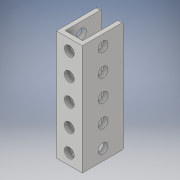
# Autodesk Inventor part: Mini Channel 5 Holes
Saved by Autodesk Inventor 2019 (Build 230136000, 136)
## iProperties
Created: 2016-08-22
Part Number: Mini Channel 5 Holes
Material: Generic
Description: STEP AP203
Document SubType Name: Modeling
Designer: mrhftc
Density: 1 g/cm^3
Appearance: Default
Sending System: SolidWorks 2014
Preprocessor: SwSTEP 2.0
Title: 585380.STEP
Revision Number: ANY
Autodesk Inventor part; units mm, degrees
ref_plane "YZ Plane" through (0, 0, 0) normal (1, 0, 0) x (0, 1, 0)
ref_plane "Work Plane1" through (4.699, 0, 1.524) normal (1, 0, 0) x (0, 0, -1)
sketch "Sketch1" plane through (4.699, 0, 1.524) normal (1, 0, 0) x (0, 0, -1)
  line L0 (-11.9322, 40.005) -> (-26.9436, 40.005)
  line L1 (-26.9436, 40.005) -> (-26.9436, 0)
  line L2 (-26.9436, 0) -> (-11.9322, 0)
  line L3 (-11.9322, 0) -> (-11.9322, 40.005)
  circle A0 centre (-19.4379, 20.0025) radius 1.778
  circle A1 centre (-19.4379, 28.0035) radius 1.778
  circle A2 centre (-19.4379, 36.0045) radius 1.778
  line L4 (-11.9322, 20.0025) -> (-25.268, 20.0025)
  circle A3 centre (-19.4379, 12.0015) radius 1.778
  circle A4 centre (-19.4379, 4.0005) radius 1.778
  point P0 (1.524, 0)
  dimension "d0" = 40.005
  dimension "d1" = 15.0114
  dimension "d2" = 3.556
  dimension "d3" = 3.556
  dimension "d4" = 3.556
  dimension "d6" = 8.001
  dimension "d7" = 8.001
  constraints: 10 end point, 5 centre point, 2 horizontal, 2 parallel, 2 symmetric about line, 1 midpoint, 1 perpendicular, 2 other
  measures "d0" distance between parallel lines of L2 L0
  measures "d1" distance between parallel lines of L1 L3
  measures "d2" diameter of A0
  measures "d3" diameter of A2
  measures "d4" diameter of A1
  measures "d6" distance of A0.centre A1.centre
  measures "d7" distance of A1.centre A2.centre
extrude "Extrusion1" add sketch "Sketch1" along normal blind 9.398
ref_plane "Work Plane2" through (4.699, 0, 13.4562) normal (0, -1, 0) x (1, 0, 0)
sketch "Sketch2" plane through (4.699, 0, 13.4562) normal (0, -1, 0) x (1, 0, 0)
  line L0 (0, 0) -> (9.398, 0) construction
  line L1 (9.398, 15.0114) -> (9.398, 0) construction
  line L2 (7.874, 13.335) -> (1.524, 13.335)
  line L3 (1.524, 13.335) -> (1.524, 0)
  line L4 (1.524, 0) -> (7.874, 0)
  line L5 (7.874, 0) -> (7.874, 13.335)
  line L6 (0, 0) -> (9.398, 0) construction
  point P0 (-4.699, -13.4562)
  dimension "d10" = 6.35
  dimension "d11" = 1.524
  dimension "d13" = 13.335
  constraints: 8 end point, 2 parallel, 1 horizontal, 1 perpendicular, 1 point on line
  measures "d10" distance between parallel lines of L3 L5
  measures "d11" distance between parallel lines of L1 L5
  measures "d13" distance between parallel lines of L2 L6
extrude "Extrusion2" cut sketch "Sketch2" against normal through all
sketch "Sketch3" plane through (4.699, 0, 28.4676) normal (0, 0, 1) x (1, 0, 0)
  circle A0 centre (4.699, 28.0103) radius 1.778
  circle A1 centre (4.699, 36.0113) radius 1.778
  circle A2 centre (4.699, 20.0093) radius 1.778
  line L0 (0, 18.2245) -> (0, 21.7805) construction
  circle A3 centre (4.699, 11.9947) radius 1.778
  circle A4 centre (4.699, 3.9937) radius 1.778
  point P0 (-4.699, 0)
  dimension "d16" = 3.556
  dimension "d17" = 3.556
  dimension "d19" = 8.001
  dimension "d20" = 8.001
  constraints: 5 centre point
  measures "d16" diameter of A1
  measures "d17" diameter of A0
  measures "d19" distance of A2.centre A0.centre
  measures "d20" distance of A0.centre A1.centre
extrude "Extrusion3" cut sketch "Sketch3" against normal through all
fillet "Fillet1" radius 0.635 4 edges at (5.461, 40.005, 13.4562) (5.461, 0, 13.4562) (13.335, 0, 13.4562) (13.335, 40.005, 13.4562)
body "Solid1"
